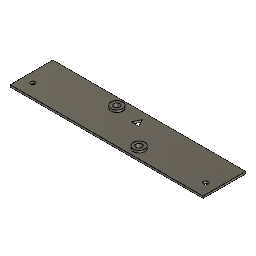
smmb_inner-bottom (Autodesk Fusion 360 design; units mm, degrees)
Autodesk Fusion 360 part; units mm, degrees
sketch "Sketch1" plane through (0, 0, 0) normal (0, 0, 1) x (1, 0, 0)
  line L0 (0, 0) -> (134, 0)
  line L1 (134, 0) -> (134, 29.874)
  line L2 (134, 29.874) -> (0, 29.874)
  line L3 (0, 29.874) -> (0, 0)
  circle A0 centre (7, 9) radius 1.55
  line L4 (67, 0) -> (67, 29.874) construction
  circle A1 centre (127, 9) radius 1.55
  line L5 (69.5, 19.874) -> (64.5, 19.874)
  line L6 (64.5, 19.874) -> (64.5, 24.874)
  line L7 (64.5, 24.874) -> (69.5, 24.874)
  line L8 (69.5, 24.874) -> (69.5, 19.874)
  line L9 (69.5, 19.874) -> (64.5, 24.874) construction
  line L10 (64.5, 19.874) -> (69.5, 24.874) construction
  line L11 (64.5, 19.874) -> (67, 24.874)
  line L12 (69.5, 19.874) -> (67, 24.874)
  point P0 (67, 22.374)
  dimension "d1" = 134
  dimension "d2" = 29.874
  dimension "d3" = 3.1
  dimension "d4" = 9
  dimension "d5" = 7
  dimension "d11" = 5
  dimension "d12" = 5
  dimension "d13" = 5
  constraint horizontal L0
  constraint vertical L1
  constraint horizontal L2
  constraint vertical L3
  constraint coincident L0.start L3.end
  constraint midpoint L0 L4.start
  constraint midpoint L2 L4.end
  constraint symmetric A0 L4 A1
  constraint perpendicular L5 L6
  constraint parallel L5 L7
  constraint parallel L6 L8
  constraint horizontal L5
  constraint coincident L9 P0
  constraint coincident L10 P0
  constraint coincident L4 P0
  constraint midpoint L7 L11.end
  measures "d1" distance of L0.start L0.end
  measures "d2" distance of L0.start L2.end
  measures "d3" diameter of A0
  measures "d4" distance of L0 A0.centre
  measures "d5" distance of L3 A0.centre
  measures "d11" distance of L5.end L6.end
  measures "d12" distance of L6.end L7.end
  measures "d13" distance of L2 L7
extrude "Extrude1" add sketch "Sketch1" along normal blind 1.5 contours L0 L1 L2 L3 | L7 L8 L12 | L6 L7 L11
sketch "Sketch2" plane through (0, 0, 1.5) normal (0, 0, 1) x (-1, 0, 0)
  circle A0 centre (-127, -9) radius 1.55
  circle A1 centre (-7, -9) radius 1.55
  line L0 (-69.5, -19.874) -> (-64.5, -19.874)
  line L1 (-64.5, -19.874) -> (-67, -24.874)
  line L2 (-67, -24.874) -> (-69.5, -19.874)
  line L3 (0, -29.874) -> (0, 0)
  line L4 (0, 0) -> (-134, 0)
  line L5 (-134, 0) -> (-134, -29.874)
  line L6 (-134, -29.874) -> (0, -29.874)
  line L7 (-67, -29.874) -> (-67, 0) construction
  line L8 (-91, -3.437) -> (-43, -3.437)
  line L9 (-43, -3.437) -> (-43, -26.437)
  line L10 (-43, -26.437) -> (-91, -26.437)
  line L11 (-91, -26.437) -> (-91, -3.437)
  line L12 (-91, -3.437) -> (-43, -26.437) construction
  line L13 (-43, -3.437) -> (-91, -26.437) construction
  circle A2 centre (-51, -23.237) radius 2.05
  circle A3 centre (-51, -23.237) radius 4.05
  circle A4 centre (-83, -6.637) radius 2.05
  circle A5 centre (-83, -6.637) radius 4.05
  point P0 (-67, -14.937)
  dimension "d14" = 48
  dimension "d15" = 23
  dimension "d18" = 8
  dimension "d19" = 3.2
  dimension "d20" = 4.1
  dimension "d21" = 8.1
  dimension "d22" = 4.1
  dimension "d23" = 8.1
  dimension "d24" = 8
  dimension "d25" = 3.2
  constraint midpoint L6 L7.start
  constraint midpoint L4 L7.end
  constraint perpendicular L8 L9
  constraint parallel L8 L10
  constraint parallel L9 L11
  constraint horizontal L8
  constraint coincident L12 P0
  constraint coincident L13 P0
  constraint midpoint L7 P0
  constraint concentric A2 A3
  constraint concentric A4 A5
  measures "d14" distance of L9.end L10.end
  measures "d15" distance of L8.end L9.end
  measures "d18" distance of L9 A2.centre
  measures "d19" distance of L10 A2.centre
  measures "d20" diameter of A2
  measures "d21" diameter of A3
  measures "d22" diameter of A4
  measures "d23" diameter of A5
  measures "d24" distance of L11 A4.centre
  measures "d25" distance of L8 A4.centre
extrude "Extrude2" add sketch "Sketch2" along normal blind 1.5 contours L8 A5 | L8 A5 | L10 A3 | L10 A3
extrude "Extrude3" cut sketch "Sketch2" against normal blind 1.5 contours A2 | A4
equation "d4 = 10.5 mm - 1.5 mm"
equation "d21 = d20 + 4 mm"
equation "d22 = d20"
equation "d23 = d21"
